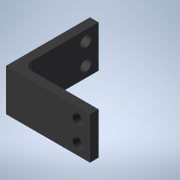
# Autodesk Inventor part: CONTROL_MONTEER
Saved by Autodesk Inventor 2020 (Build 240168000, 168)
## iProperties
Created: 2020-06-03
Part Number: CONTROL_MONTEER
Material: Generic
Document SubType Name: Modeling
Designer: Gebruiker
Density: 1 g/cm^3
Appearance: Default
Author: Gebruiker
Autodesk Inventor part; units mm, degrees
ref_plane "YZ Plane" through (0, 0, 0) normal (1, 0, 0) x (0, 1, 0)
ref_plane "XZ Plane" through (0, 0, 0) normal (0, 1, 0) x (-1, 0, 0)
ref_plane "XY Plane" through (0, 0, 0) normal (0, 0, 1) x (1, 0, 0)
sketch "Sketch1" plane through (0, 0, 0) normal (0, 0, 1) x (1, 0, 0)
  line L0 (-10, 5) -> (10, 5)
  line L1 (10, 5) -> (10, -5)
  line L2 (10, -5) -> (-10, -5)
  line L3 (-10, -5) -> (-10, 5)
  line L4 (-10, 5) -> (10, -5) construction
  line L5 (10, 5) -> (-10, -5) construction
  point P0 (0, 0)
  dimension "d0" = 20
  dimension "d1" = 10
  constraints: 12 end point, 2 midpoint, 2 parallel, 1 horizontal, 1 perpendicular
  measures "d0" distance of L1.end L2.end
  measures "d1" distance of L0.end L1.end
extrude "Extrusion1" add sketch "Sketch1" against normal blind 2
sketch "Sketch2" plane through (-10, 5, 0) normal (0, 1, 0) x (1, 0, 0)
  line L0 (20, 0) -> (0, 0) projected
  line L1 (0, 0) -> (2, 0)
  line L2 (2, 0) -> (2, 20)
  line L3 (2, 20) -> (0, 20)
  line L4 (0, 20) -> (0, 0)
  point P0 (10, 0)
  point P1 (2, 0)
  dimension "d4" = 2
  dimension "d5" = 20
  constraints: 8 end point, 2 parallel, 1 horizontal, 1 perpendicular
  measures "d4" distance of L3.end L2.end
  measures "d5" distance of L2.end L1.end
extrude "Extrusion2" add sketch "Sketch2" against normal blind 10
fillet "Fillet1" radius 2 1 edges at (-8, 0, -2)
sketch "Sketch4" plane through (0, 0, -2) normal (0, 0, -1) x (-1, 0, 0)
  circle A0 centre (-7, -2.5) radius 1.25
  circle A1 centre (-7, 2.5) radius 1.25
  line L0 (-10, -5) -> (6, -5) projected
  line L1 (6, 5) -> (-10, 5) projected
  line L2 (-10, 5) -> (-10, -5) projected
  point P0 (0, 0)
  dimension "d10" = 2.5
  dimension "d11" = 2.5
  dimension "d12" = 2.5
  dimension "d13" = 2.5
  dimension "d15" = 3
  dimension "d16" = 3
  constraints: 2 centre point
  measures "d10" diameter of A0
  measures "d11" diameter of A1
  measures "d12" distance from line of A0.centre L0
  measures "d13" distance from line of L1 A1.centre
  measures "d15" distance from line of L2 A1.centre
  measures "d16" distance from line of L2 A0.centre
extrude "Extrusion3" cut sketch "Sketch4" against normal blind 2
sketch "Sketch5" plane through (-8, -5, -20) normal (1, 0, 0) x (0, 0, -1)
  circle A0 centre (-3, 2.5) radius 1.25
  circle A1 centre (-3, 7.5) radius 1.25
  line L0 (0, 0) -> (-16, 0) projected
  line L1 (-16, 10) -> (0, 10) projected
  line L2 (0, 10) -> (0, 0) projected
  point P0 (-20, 5)
  dimension "d19" = 2.5
  dimension "d20" = 2.5
  dimension "d21" = 2.5
  dimension "d22" = 2.5
  dimension "d23" = 3
  dimension "d24" = 3
  constraints: 2 centre point
  measures "d19" diameter of A0
  measures "d20" diameter of A1
  measures "d21" distance from line of A0.centre L0
  measures "d22" distance from line of L1 A1.centre
  measures "d23" distance from line of L2 A1.centre
  measures "d24" distance from line of L2 A0.centre
extrude "Extrusion4" cut sketch "Sketch5" against normal blind 2
body "Solid1"
